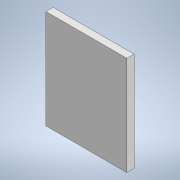
# Autodesk Inventor part: PCB_2
Saved by Autodesk Inventor 2022 (Build 260153000, 153)
## iProperties
Created: 2022-12-27
Part Number: PCB_2
Material: Generic
Document SubType Name: Modeling
Designer: Kamil
Density: 1 g/cm^3
Appearance: Default
Author: Kamil
Autodesk Inventor part; units mm, degrees
ref_plane "YZ Plane" through (0, 0, 0) normal (1, 0, 0) x (0, 1, 0)
ref_plane "XZ Plane" through (0, 0, 0) normal (0, 1, 0) x (-1, 0, 0)
ref_plane "XY Plane" through (0, 0, 0) normal (0, 0, 1) x (1, 0, 0)
sketch "Sketch1" plane through (0, 0, 0) normal (0, 0, 1) x (1, 0, 0)
  circle A0 centre (7.5, -12.2) radius 1.75 projected
  circle A1 centre (-7.5, -12.2) radius 1.75 projected
  line L0 (-15, -5.24) -> (-12.5, -5.24) projected
  arc A2 (-12.5, -10.24) -> (-12.5, -5.24) centre (-12.5, -7.74) ccw projected
  line L1 (-12.5, -10.24) -> (-15, -10.24) projected
  line L2 (-15, -10.24) -> (-15, -5.24) projected
  line L3 (12.5, -5.24) -> (15, -5.24) projected
  line L4 (15, -5.24) -> (15, -10.24) projected
  line L5 (15, -10.24) -> (12.5, -10.24) projected
  arc A3 (12.5, -5.24) -> (12.5, -10.24) centre (12.5, -7.74) ccw projected
  line L6 (37.5, -15.4) -> (37.5, 31.2121) projected
  line L7 (37.5, 31.2121) -> (14.8602, 31.2121) projected
  line L8 (14.8602, 31.2121) -> (14.8602, 15.1552) projected
  line L9 (14.8602, 15.1552) -> (2.8777, -5.8186) projected
  line L10 (2.8777, -5.8186) -> (-2.8777, -5.8186) projected
  line L11 (-2.8777, -5.8186) -> (-15, 15.4) projected
  line L12 (-15, 15.4) -> (-15, 31.2121) projected
  line L13 (-15, 31.2121) -> (-37.5, 31.2121) projected
  line L14 (-37.5, 31.2121) -> (-37.5, -15.4) projected
  line L15 (-37.5, -15.4) -> (37.5, -15.4) projected
  line L16 (44, 22.1656) -> (44, -5.24) projected
  line L17 (44, 3.8199) -> (40.2471, -6.356) projected
  line L18 (40.2471, -9.1241) -> (44, -19.3) projected
  line L19 (50, 15.6109) -> (-50, 15.6109) projected
  line L20 (50, 15.6109) -> (-50, 15.6109) projected
  line L21 (-14.8795, 22.2639) -> (-42.2795, 22.2397) projected
  line L22 (-21.0553, -5.1415) -> (-14.8553, -5.136) projected
  line L23 (17.7513, -5.24) -> (37.5, -5.24)
  line L24 (37.5, -5.24) -> (37.5, 22.3103)
  line L25 (37.5, 22.3103) -> (17.7513, 22.3103)
  line L26 (17.7513, 22.3103) -> (17.7513, -5.24)
  line L27 (37.5, 22.3103) -> (15, 22.3103)
  line L28 (15, 22.3103) -> (15, -5.24)
  line L29 (15, -5.24) -> (37.5, -5.24)
  line L30 (37.5, -5.24) -> (37.5, 22.3103)
  point P0 (0, 0)
  constraints: 16 end point, 4 parallel, 2 horizontal, 2 perpendicular, 1 point on line
extrude "Extrusion1" add sketch "Sketch1" along normal blind 2.4 contours L28 L19 L26 L29 | L28 L27 L26 L19 | L26 L19 L6 L23 | L26 L25 L6 L19
sketch "Sketch2" plane through (0, 0, 0) normal (0, 0, -1) x (-1, 0, 0)
  line L0 (-15, -5.24) -> (-37.5, -5.24) projected
  line L1 (-37.5, -5.24) -> (-37.5, 22.3103) projected
  line L2 (-37.5, 22.3103) -> (-15, 22.3103) projected
  line L3 (-15, 22.3103) -> (-15, -5.24) projected
  point P0 (0, 0)
extrude "Extrusion2" cut sketch "Sketch2" against normal blind 0.4
sketch "Sketch3" plane through (0, 0, 2.4) normal (0, 0, 1) x (1, 0, 0)
  line L0 (15, -5.24) -> (37.5, -5.24) projected
  line L1 (37.5, -5.24) -> (37.5, 22.3103) projected
  line L2 (37.5, 22.3103) -> (15, 22.3103) projected
  line L3 (15, 22.3103) -> (15, -5.24) projected
  circle A0 centre (7.5, -12.2) radius 1.75 projected
  circle A1 centre (-7.5, -12.2) radius 1.75 projected
  line L4 (-15, -5.24) -> (-12.5, -5.24) projected
  arc A2 (-12.5, -10.24) -> (-12.5, -5.24) centre (-12.5, -7.74) ccw projected
  line L5 (-12.5, -10.24) -> (-15, -10.24) projected
  line L6 (-15, -10.24) -> (-15, -5.24) projected
  line L7 (12.5, -5.24) -> (15, -5.24) projected
  line L8 (15, -5.24) -> (15, -10.24) projected
  line L9 (15, -10.24) -> (12.5, -10.24) projected
  arc A3 (12.5, -5.24) -> (12.5, -10.24) centre (12.5, -7.74) ccw projected
  line L10 (37.5, -15.4) -> (37.5, 31.2121) projected
  line L11 (37.5, 31.2121) -> (14.8602, 31.2121) projected
  line L12 (14.8602, 31.2121) -> (14.8602, 15.1552) projected
  line L13 (14.8602, 15.1552) -> (2.8777, -5.8186) projected
  line L14 (2.8777, -5.8186) -> (-2.8777, -5.8186) projected
  line L15 (-2.8777, -5.8186) -> (-15, 15.4) projected
  line L16 (-15, 15.4) -> (-15, 31.2121) projected
  line L17 (-15, 31.2121) -> (-37.5, 31.2121) projected
  line L18 (-37.5, 31.2121) -> (-37.5, -15.4) projected
  line L19 (-37.5, -15.4) -> (37.5, -15.4) projected
  line L20 (37.5, -5.24) -> (15, -5.24)
  line L21 (15, -5.24) -> (15, -15.4)
  line L22 (15, -15.4) -> (37.5, -15.4)
  line L23 (37.5, -15.4) -> (37.5, -5.24)
  point P0 (0, 0)
  constraints: 8 end point, 2 parallel, 1 horizontal, 1 perpendicular, 1 point on line
extrude "Extrusion3" add sketch "Sketch3" against normal blind 2 contours L0 L10 L19 L21 L8
body "Solid1"
